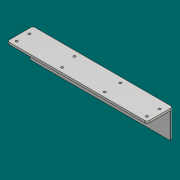
# Autodesk Inventor part: kpd_70_cover
Saved by Autodesk Inventor 2018 (Build 220112000, 112)
## iProperties
Created: 2022-01-26
Part Number: kpd_70_cover
Material: アルミニウム 6061
Document SubType Name: Modeling
Designer: gisen
Density: 2.7 g/cm^3
Appearance: アルミニウム - フラット
Author: gisen
Autodesk Inventor part; units mm, degrees
ref_plane "YZ Plane" through (0, 0, 0) normal (1, 0, 0) x (0, 1, 0)
ref_plane "XZ Plane" through (0, 0, 0) normal (0, 1, 0) x (-1, 0, 0)
ref_plane "XY Plane" through (0, 0, 0) normal (0, 0, 1) x (1, 0, 0)
sketch "スケッチ1" plane through (0, 0, 0) normal (0, 0, 1) x (1, 0, 0)
  line L0 (-120.5, 11.775) -> (120.5, 11.775) construction
  line L1 (120.5, 11.775) -> (120.5, -11.775) construction
  line L2 (120.5, -11.775) -> (-120.5, -11.775) construction
  line L3 (-120.5, -11.775) -> (-120.5, 11.775) construction
  circle A0 centre (-120.5, -11.775) radius 2.25
  circle A1 centre (-120.5, 11.775) radius 2.25
  circle A2 centre (-36.5, -11.775) radius 2.25
  circle A3 centre (42.5, -11.775) radius 2.25
  circle A4 centre (120.5, -11.775) radius 2.25
  line L4 (-129.5, 22.275) -> (-129.5, -20.275) construction
  line L5 (-129.5, 22.275) -> (129.5, 22.275) construction
  line L6 (129.5, 22.275) -> (129.5, -20.275) construction
  line L7 (129.5, -20.275) -> (-129.5, -20.275) construction
  circle A5 centre (-42.5, 17.275) radius 2.25
  circle A6 centre (42.5, 17.275) radius 2.25
  circle A7 centre (120.5, 11.775) radius 2.25
  line L8 (-129.5, -20.275) -> (129.5, -20.275)
  line L9 (129.5, -20.275) -> (129.5, 27.275)
  line L10 (129.5, 27.275) -> (-129.5, 27.275)
  line L11 (-129.5, 27.275) -> (-129.5, -20.275)
  point P0 (0, 0)
  point P1 (-120.5, 0)
  point P2 (0, 11.775)
  dimension "d0" = 23.55
  dimension "d1" = 84
  dimension "d3" = 79
  dimension "d4" = 78
  dimension "d5" = 4.5
  dimension "d6" = 9
  dimension "d7" = 9
  dimension "d8" = 8.5
  dimension "d9" = 10.5
  dimension "d10" = 5.5
  dimension "d11" = 78.1937
  dimension "d12" = 78.1937
  dimension "d13" = 78
  dimension "d14" = 85
  dimension "d15" = 78
  dimension "d16" = 5
  constraints: 24 end point, 8 centre point, 8 coincident, 7 equal radius, 4 parallel, 4 perpendicular, 3 horizontal, 2 horizontal alignment, 2 midpoint, 2 point on line, 1 vertical, 1 vertical alignment
  measures "d0" distance of L2.end L0.start
  measures "d1" distance of point (-36.5, -11.775) L2.end
  measures "d3" distance of point (42.5, -11.775) point (-36.5, -11.775)
  measures "d4" distance from line of L1 point (42.5, -11.775)
  measures "d5" diameter of A0
  measures "d6" distance between parallel lines of L3 L4
  measures "d7" distance between parallel lines of L6 L1
  measures "d8" distance between parallel lines of L7 L2
  measures "d9" distance between parallel lines of L0 L5
  measures "d10" distance from line of L0 point (-42.5, 17.275)
  measures "d11" distance of point (-42.5, 17.275) L0.start
  measures "d12" distance of L0.end point (42.5, 17.275)
  measures "d13" horizontal distance of point (-42.5, 17.275) L0.start
  measures "d14" distance of point (42.5, 17.275) point (-42.5, 17.275)
  measures "d15" horizontal distance of L0.end A6.centre
  measures "d16" distance between parallel lines of L5 L10
extrude "押し出し1" add sketch "スケッチ1" along normal blind 4
sketch "スケッチ2" plane through (0, 0, 0) normal (0, 0, -1) x (-1, 0, 0)
  line L0 (129.5, 22.275) -> (-129.5, 22.275) construction
  line L1 (-129.5, 22.275) -> (129.5, 22.275)
  line L2 (129.5, 22.275) -> (129.5, 27.275)
  line L3 (129.5, 27.275) -> (-129.5, 27.275)
  line L4 (-129.5, 27.275) -> (-129.5, 22.275)
  line L5 (-129.5, 27.275) -> (129.5, 27.275) construction
  point P0 (0, 0)
  constraints: 8 end point, 2 parallel, 1 horizontal, 1 perpendicular
extrude "押し出し2" add sketch "スケッチ2" along normal blind 47.4
fillet "フィレット1" radius 4 2 edges at (-129.5, -20.275, 2) (129.5, -20.275, 2)
fillet "フィレット2" [suppressed]
fillet "フィレット3" radius 4 2 edges at (129.5, 27.275, -21.7) (-129.5, 27.275, -21.7)
equation "\"d12\" = d11"
